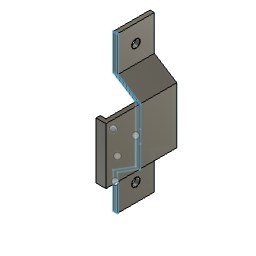
cooling_plate_bracket v10 (Autodesk Fusion 360 design; units mm, degrees)
Autodesk Fusion 360 part; units mm, degrees
note: some values were not read from the file. Set by a fixed rule: which face or edge a step refers to.
sketch "Sketch1" plane through (0, 0, 0) normal (0, 1, 0) x (1, 0, 0) in component "Bracket"
  line L0 (0, 10) -> (0, 35)
  line L1 (0, 10) -> (15.875, 0)
  line L2 (0, -49.7) -> (15.875, -39.7)
  line L3 (0, -49.7) -> (0, -74.7)
  line L4 (3, 10) -> (18.875, 0)
  line L5 (3, -49.7) -> (3, -74.7)
  line L6 (3, 10) -> (3, 35)
  line L7 (3, -49.7) -> (18.875, -39.7)
  line L8 (0, -74.7) -> (3, -74.7)
  line L9 (0, 35) -> (3, 35)
  line L10 (3, 16.3237) -> (1.5, 16.3237)
  line L11 (15.875, 0) -> (15.875, -18.9765)
  line L12 (15.875, 0) -> (15.875, -16.7759)
  line L13 (15.875, -16.7759) -> (15.875, -39.7)
  line L14 (18.875, 0) -> (18.875, -15.35)
  line L15 (18.875, -24.35) -> (18.875, -39.7)
  line L16 (18.875, -15.35) -> (18.875, -24.35)
  point P0 (3, 0)
  dimension "d5" = 25
  dimension "d7" = 25
  dimension "d8" = 25
  dimension "d9" = 25
  constraint vertical L0
  constraint vertical L6
  constraint perpendicular L5 L8
  constraint perpendicular L6 L9
  constraint coincident L6 L10.start
  constraint perpendicular L10 L12
  constraint parallel L11 L12
  constraint collinear L12 L13
  constraint collinear L14 L15
  constraint parallel L15 L16
  measures "d5" distance of L0.start L0.end
  measures "d7" distance of L2.start L3.end
  measures "d8" distance of L4.start L6.end
  measures "d9" distance of L5.end L5.start
sketch "Sketch4" plane through (0, 0, 0) normal (0, 1, 0) x (1, 0, 0) in component "Bracket"
extrude "Extrude4" add sketch "Sketch1" along normal blind 26 makes body 1 in component "Bracket"
hole "Hole6" at (3, 13, -22.5) direction (-1, 0, 0) diameter 6 depth 30 tip angle 118 bodies 1 in component "Bracket"
hole "Hole7" at (3, 13, 62.2) direction (-1, 0, 0) diameter 6 depth 30 tip angle 118 bodies 1 in component "Bracket"
extrude "Extrude3" add sketch "Sketch1" along normal blind 26 separate body makes body 2 in component "Bracket"
sketch "Sketch3" plane through (0, 0, 0) normal (1, 0, 0) x (0, 1, 0) in component "Bracket"
  spline S0 degree 5 poles (0, 15) (0, 14.9529) (0, 14.864) (0, 14.7459) (0, 14.6199) (0, 14.5181) (0, 14.4763) (0, 14.4987) (0, 14.5857) (0, 14.7331) (0, 14.9358) (0, 15.1381) (0, 15.311) (0, 15.4355) (0, 15.5) knots 0 0 0 0 0 0 0.1 0.2 0.3 0.4 0.5 0.6 0.7 0.8 0.9 1 1 1 1 1 1
  point P0 (0, 14.5)
extrude "Extrude2" add sketch "Sketch1" along normal blind 26 separate body makes body 3 in component "Bracket"
sketch "Sketch1 (2)" plane through (0, 26, 0) normal (0, 1, 0) x (-1, 0, 0)
  line L0 (-3, -10) -> (-3, -35)
  line L1 (-3, -35) -> (0, -35)
  line L2 (0, -35) -> (0, -10)
  line L3 (0, -10) -> (-15.875, 0)
  line L4 (-15.875, 0) -> (-15.875, 39.7)
  line L5 (-15.875, 39.7) -> (0, 49.7)
  line L6 (0, 49.7) -> (0, 74.7)
  line L7 (0, 74.7) -> (-3, 74.7)
  line L8 (-3, 74.7) -> (-3, 49.7)
  line L9 (-3, 49.7) -> (-18.875, 39.7)
  line L10 (-18.875, 39.7) -> (-18.875, 0)
  line L11 (-18.875, 0) -> (-3, -10)
  line L12 (-18.875, 39.7, -26) -> (-18.875, 39.7, -47)
  line L13 (-18.875, 0, -26) -> (-18.875, 0, -47)
  line L14 (-18.875, 39.7, -47) -> (-18.875, 0, -47)
  line L15 (-18.875, 39.7, -26) -> (-18.875, 0, -26)
  point P0 (-18.875, 39.7)
  point P1 (-18.875, 0)
  dimension "d63" = 21
  dimension "d64" = 21
  constraint coincident P0 L9.end
  constraint coincident P1 L10.end
  measures "d63" distance of P0 L9.end
  measures "d64" distance of P1 L10.end
extrude "Extrude1" add sketch "Sketch1 (2)" along normal blind 3 separate body contours L12 L13 L14 L15 in plane through (18.875, 26, 0) normal (-1, 0, 0) makes body 4
sketch "Sketch2" plane through (15.875, 0, 0) normal (-1, 0, 0) x (0, -1, 0)
  line L0 (21, 39.7) -> (0, 39.7)
  line L1 (0, 39.7) -> (0, 0)
  line L2 (0, 0) -> (21, 0)
  line L3 (21, 0) -> (21, 39.7)
  line L4 (21, 39.7, -3) -> (21, 39.7, 4)
  line L5 (21, 0, -3) -> (21, 0, 4)
  line L6 (21, 39.7, 4) -> (21, 0, 4)
  line L7 (21, 39.7, -3) -> (21, 0, -3)
  point P0 (21, 39.7)
  point P1 (21, 0)
  dimension "d67" = 7
  dimension "d68" = 7
  constraint coincident P0 L0.start
  constraint coincident P1 L2.end
  measures "d67" distance of P0 L0.start
  measures "d68" distance of P1 L2.end
extrude "Extrude2'" add sketch "Sketch2" along normal blind 3 separate body contours L3 L4 L5 L6 in plane through (15.875, -21, 0) normal (0, -1, 0) makes body 5
extrude "Extrude3'" add 1 faces at (17.875, -21, 26.4667) along direction (0, -1, 0) blind 3 on bodies 4 bodies 4 5
sketch "Sketch3 (2)" plane through (0, 26, 0) normal (0, 1, 0) x (-1, 0, 0)
  line L0 (-3, -10) -> (-3, -35)
  line L1 (-3, -35) -> (0, -35)
  line L2 (0, -35) -> (0, -10)
  line L3 (0, -10) -> (-15.875, 0)
  line L4 (-15.875, 0) -> (-15.875, 39.7)
  line L5 (-15.875, 39.7) -> (0, 49.7)
  line L6 (0, 49.7) -> (0, 74.7)
  line L7 (0, 74.7) -> (-3, 74.7)
  line L8 (-3, 74.7) -> (-3, 49.7)
  line L9 (-3, 49.7) -> (-18.875, 39.7)
  line L10 (-18.875, 39.7) -> (-18.875, 0)
  line L11 (-18.875, 0) -> (-3, -10)
hole "Hole8" at (3, 13, -22.5) direction (-1, 0, 0) diameter 5.5 depth 22 tip angle 118 bodies 2 3 in component "Bracket"
hole "Hole9" at (3, 13, 62.2) direction (-1, 0, 0) diameter 5.5 depth 22 tip angle 118 bodies 2 3 in component "Bracket"
hole "Hole3" [rolled back] hole depth 30 hole diameter 6 tip angle 118 in component "Bracket"
hole "Hole4" [rolled back] hole depth 30 hole diameter 6 tip angle 118 ref dim1 12.5 ref dim2 13 in component "Bracket"
hole "Hole5" [rolled back] hole depth 30 hole diameter 6 tip angle 118 ref dim1 12.5 ref dim2 13 in component "Bracket"
extrude "Extrude1'" [rolled back] along distance 26 taper angle 0 in component "Bracket"
hole "Hole1" [rolled back] hole depth 10 hole diameter 5 tip angle 118 ref dim1 13 ref dim2 12.5 in component "Bracket"
hole "Hole2" [rolled back] hole depth 10 hole diameter 5 tip angle 118 ref dim1 13 ref dim2 12.5 in component "Bracket"
sketch "Sketch2 (2)" plane through (0, 0, 0) normal (0, 1, 0) x (1, 0, 0) in component "Bracket"
component "Bracket" placed x (1, 0, 0) y (0, 1, 0) z (0, 0, 1) at (0, 0, 0)
